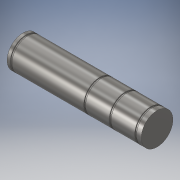
# Autodesk Inventor part: Center Axle
Saved by Autodesk Inventor 2019.4 (Build 234330000, 330)
## iProperties
Created: 2019-12-14
Part Number: Center Axle
Material: Steel, Mild
Document SubType Name: Modeling
Designer: admin
Density: 7.85 g/cm^3
Appearance: Semi-Polished
Author: admin
Autodesk Inventor part; units mm, degrees
ref_plane "YZ Plane" through (0, 0, 0) normal (1, 0, 0) x (0, 1, 0)
ref_plane "XZ Plane" through (0, 0, 0) normal (0, 1, 0) x (-1, 0, 0)
ref_plane "XY Plane" through (0, 0, 0) normal (0, 0, 1) x (1, 0, 0)
sketch "Sketch1" plane through (0, 0, 0) normal (0, 0, 1) x (1, 0, 0)
  line L0 (64.6, 10) -> (64.6, 9.5)
  line L1 (64.6, 9.5) -> (65.7, 9.5)
  line L2 (65.7, 9.5) -> (65.7, 10)
  line L3 (65.7, 10) -> (80.7, 10)
  line L4 (80.7, 10) -> (80.7, 9.5)
  line L5 (80.7, 9.5) -> (81.8, 9.5)
  line L6 (81.8, 9.5) -> (81.8, 10)
  line L7 (81.8, 10) -> (84.8, 10)
  line L8 (84.8, 10) -> (84.8, 0)
  line L9 (84.8, 0) -> (0, 0)
  line L10 (0, 10) -> (0, 0)
  line L11 (64.6, 10) -> (49.6, 10)
  line L12 (49.6, 10) -> (49.6, 9.5)
  line L13 (49.6, 9.5) -> (48.5, 9.5)
  line L14 (48.5, 9.5) -> (48.5, 10)
  line L15 (0, 10) -> (2, 10)
  line L16 (2, 10) -> (2, 9.5)
  line L17 (2, 9.5) -> (3.1, 9.5)
  line L18 (3.1, 9.5) -> (3.1, 10)
  line L19 (3.1, 10) -> (48.5, 10)
  dimension "d3" = 1.1
  dimension "d5" = 1.1
  dimension "d6" = 10
  dimension "d12" = 3
  dimension "d20" = 0.5
  dimension "d21" = 0.5
  dimension "d22" = 0.5
  dimension "d23" = 15
  dimension "d32" = 64.6
  dimension "d33" = 15
  dimension "d34" = 1.1
  dimension "d35" = 0.5
  dimension "d36" = 1.1
  dimension "d37" = 0.5
  dimension "d38" = 2
  constraints: 40 end point, 13 perpendicular, 6 point on line, 3 horizontal, 1 vertical
  measures "d3" distance of L0.end L1.end
  measures "d5" distance of L4.end L5.end
  measures "d6" distance between parallel lines of L9 L3
  measures "d12" distance of L6.end L7.end
  measures "d20" distance of L0.start L0.end
  measures "d21" distance of L3.end L4.end
  measures "d22" distance of L1.end L2.end
  measures "d23" distance of L2.end L3.end
  measures "d32" distance of L10.start L0.start
  measures "d33" distance of L0.start L11.end
  measures "d34" distance of L12.end L13.end
  measures "d35" distance of L11.end L12.end
  measures "d36" distance of L16.end L17.end
  measures "d37" distance of L15.end L16.end
  measures "d38" distance of L10.start L15.end
revolve "Revolution1" add sketch "Sketch1" angle 360 about axis through (84.8, 0, 0) along (-1, 0, 0)
sketch "Sketch2" plane through (43, 0, 0) normal (1, 0, 0) x (0, 0, -1)
  arc A0 (19.9153, -3.9332) -> (19.9669, 3.6623) centre (0, 0) ccw projected
  arc A1 (20.9085, 5.1405) -> (19.9669, 3.6623) centre (21.2333, 3.8946) ccw projected
  line L0 (20.9085, 5.1405) -> (23.1638, 5.7284) projected
  arc A2 (24.7533, 4.7239) -> (23.1638, 5.7284) centre (23.4886, 4.4826) ccw projected
  arc A3 (24.6868, -5.0596) -> (24.7533, 4.7239) centre (0, 0) ccw projected
  arc A4 (23.0839, -6.0425) -> (24.6868, -5.0596) centre (23.4256, -4.8011) ccw projected
  line L1 (23.0839, -6.0425) -> (20.8368, -5.424) construction
  arc A5 (19.9153, -3.9332) -> (20.8368, -5.424) centre (21.1784, -4.1826) ccw projected
  circle A6 centre (20.5409, -12.046) radius 2.1526 construction
  arc A7 (25.2444, 4.8176) -> (23.0377, 6.2122) centre (23.4886, 4.4826) ccw
  line L2 (23.0377, 6.2122) -> (20.7824, 5.6243)
  arc A8 (20.7824, 5.6243) -> (19.4751, 3.5721) centre (21.2333, 3.8946) ccw
  arc A9 (19.4248, -3.8363) -> (19.4751, 3.5721) centre (0, 0) ccw
  arc A10 (19.4248, -3.8363) -> (20.7041, -5.906) centre (21.1784, -4.1826) ccw
  line L3 (20.7041, -5.906) -> (22.9512, -6.5245)
  arc A11 (22.9512, -6.5245) -> (25.1767, -5.16) centre (23.4256, -4.8011) ccw
  arc A12 (25.1767, -5.16) -> (25.2444, 4.8176) centre (0, 0) ccw
  circle A13 centre (20.5409, -12.046) radius 2.6526
  arc A14 (17.126, 16.6141) -> (17.057, 19.2236) centre (15.8707, 17.8866) ccw
  line L4 (15.4668, 14.9772) -> (17.126, 16.6141)
  arc A15 (13.0347, 14.9042) -> (15.4668, 14.9772) centre (14.2115, 16.2497) ccw
  arc A16 (13.0347, 14.9042) -> (6.644, 18.652) centre (0, 0) ccw
  arc A17 (5.5204, 20.8102) -> (6.644, 18.652) centre (7.2438, 20.3359) ccw
  line L5 (6.1389, 23.0574) -> (5.5204, 20.8102)
  arc A18 (8.45, 24.2711) -> (6.1389, 23.0574) centre (7.8623, 22.583) ccw
  arc A19 (17.057, 19.2236) -> (8.45, 24.2711) centre (0, 0) ccw
  circle A20 centre (20.7026, 11.7659) radius 2.6526
  arc A21 (-5.8252, 23.1386) -> (-8.1196, 24.3836) centre (-7.5549, 22.6877) ccw
  line L6 (-5.2373, 20.8833) -> (-5.8252, 23.1386)
  arc A22 (-6.3901, 18.7405) -> (-5.2373, 20.8833) centre (-6.967, 20.4324) ccw
  arc A23 (-6.3901, 18.7405) -> (-12.8311, 15.0799) centre (0, 0) ccw
  arc A24 (-15.262, 15.1859) -> (-12.8311, 15.0799) centre (-13.9895, 16.4412) ccw
  line L7 (-16.8988, 16.8451) -> (-15.262, 15.1859)
  arc A25 (-16.7944, 19.4535) -> (-16.8988, 16.8451) centre (-15.6263, 18.1004) ccw
  arc A26 (-8.1196, 24.3836) -> (-16.7944, 19.4535) centre (0, 0) ccw
  circle A27 centre (0.1617, 23.812) radius 2.6526
  arc A28 (-22.9512, 6.5245) -> (-25.1767, 5.16) centre (-23.4256, 4.8011) ccw
  line L8 (-20.7041, 5.906) -> (-22.9512, 6.5245)
  arc A29 (-19.4248, 3.8363) -> (-20.7041, 5.906) centre (-21.1784, 4.1826) ccw
  arc A30 (-19.4248, 3.8363) -> (-19.4751, -3.5721) centre (0, 0) ccw
  arc A31 (-20.7824, -5.6243) -> (-19.4751, -3.5721) centre (-21.2333, -3.8946) ccw
  line L9 (-23.0377, -6.2122) -> (-20.7824, -5.6243)
  arc A32 (-25.2444, -4.8176) -> (-23.0377, -6.2122) centre (-23.4886, -4.4826) ccw
  arc A33 (-25.1767, 5.16) -> (-25.2444, -4.8176) centre (0, 0) ccw
  circle A34 centre (-20.5409, 12.046) radius 2.6526
  arc A35 (-17.126, -16.6141) -> (-17.057, -19.2236) centre (-15.8707, -17.8866) ccw
  line L10 (-15.4668, -14.9772) -> (-17.126, -16.6141)
  arc A36 (-13.0347, -14.9042) -> (-15.4668, -14.9772) centre (-14.2115, -16.2497) ccw
  arc A37 (-13.0347, -14.9042) -> (-6.644, -18.652) centre (0, 0) ccw
  arc A38 (-5.5204, -20.8102) -> (-6.644, -18.652) centre (-7.2438, -20.3359) ccw
  line L11 (-6.1389, -23.0574) -> (-5.5204, -20.8102)
  arc A39 (-8.45, -24.2711) -> (-6.1389, -23.0574) centre (-7.8623, -22.583) ccw
  arc A40 (-17.057, -19.2236) -> (-8.45, -24.2711) centre (0, 0) ccw
  circle A41 centre (-20.7026, -11.7659) radius 2.6526
  arc A42 (5.8252, -23.1386) -> (8.1196, -24.3836) centre (7.5549, -22.6877) ccw
  line L12 (5.2373, -20.8833) -> (5.8252, -23.1386)
  arc A43 (6.3901, -18.7405) -> (5.2373, -20.8833) centre (6.967, -20.4324) ccw
  arc A44 (6.3901, -18.7405) -> (12.8311, -15.0799) centre (0, 0) ccw
  arc A45 (15.262, -15.1859) -> (12.8311, -15.0799) centre (13.9895, -16.4412) ccw
  line L13 (16.8988, -16.8451) -> (15.262, -15.1859)
  arc A46 (16.7944, -19.4535) -> (16.8988, -16.8451) centre (15.6263, -18.1004) ccw
  arc A47 (8.1196, -24.3836) -> (16.7944, -19.4535) centre (0, 0) ccw
  circle A48 centre (-0.1617, -23.812) radius 2.6526
  point P0 (0, 0)
  dimension "d24" = 0.5
  dimension "d25" = 0.5
  dimension "d28" = 360
  constraints: 72 point on circle, 42 centre point, 24 end point, 152 other
  measures "d24" radial gap between concentric circles of A3 A12
  measures "d25" radial gap between concentric circles of A6 A13
extrude "Extrusion1" [suppressed]
body "Solid1"
